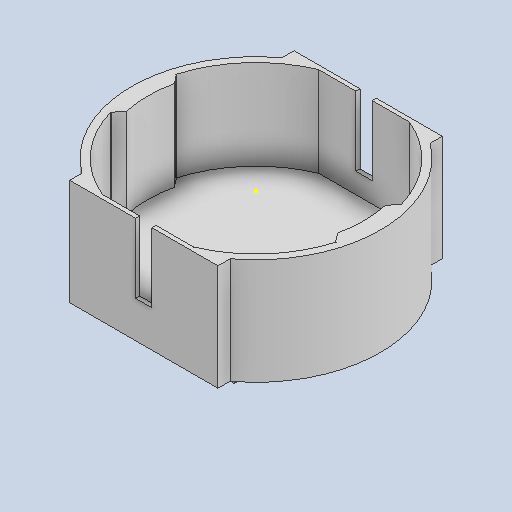
# Autodesk Inventor part: BigLif2
Saved by Autodesk Inventor 2025 (Build 290162000, 162)
## iProperties
Created: 2025-08-07
Part Number: BigLif2
Material: Generic
Document SubType Name: Modeling
Designer: Pravoslav
Density: 1 g/cm^3
Appearance: Default
Author: Pravoslav
Autodesk Inventor part; units mm, degrees
sketch "Sketch1" plane through (0, 0, 0) normal (0, 1, 0) x (-1, 0, 0)
  circle A0 centre (0, 0) radius 26.5
  circle A1 centre (0, 0) radius 30.5
  dimension "d0" = 53
  dimension "d1" = 4
  constraints: 2 centre point, 2 coincident
  measures "d0" diameter of A0
  measures "d1" radial gap between concentric circles of A0 A1
extrude "Extrusion1" add sketch "Sketch1" along normal blind 22
extrude "Extrusion2" add sketch "Sketch1" against normal blind 4 contours A0 | A1
ref_plane "Work Plane1" through (0, 15, 0) normal (0, 1, 0) x (1, 0, 0)
ref_plane "Work Plane2" through (30.5, 0, 0) normal (1, 0, 0) x (0, 1, 0)
sketch "Sketch3" plane through (30.5, 0, 0) normal (1, 0, 0) x (0, 1, 0)
  line L0 (14, -18.4883) -> (14, 18.4883) projected
  line L1 (16, 18.4883) -> (16, -18.4883) projected
  line L2 (16, 21.067) -> (16, 18.4883) projected
  line L3 (14, 18.4883) -> (14, 21.067) projected
  line L4 (16, 21.067) -> (16, -21.067) projected
  line L5 (16, 21.067) -> (16, 18.4883) projected
  line L6 (16, 18.4883) -> (16, -18.4883) projected
  line L7 (16, -18.4883) -> (16, -21.067) projected
  line L8 (14, -21.067) -> (14, -18.4883) projected
  line L9 (23, 32.2933) -> (-6, 32.2933)
  line L10 (-6, 32.2933) -> (-6, -38.454)
  line L11 (-6, -38.454) -> (23, -38.454)
  line L12 (23, -38.454) -> (23, 32.2933)
  line L13 (23, 24.5) -> (-6, 24.5)
  line L14 (23, -24.5) -> (-6.5731, -24.5)
  line L15 (-4, 30.5) -> (22, 30.5) projected
  line L16 (-4, -30.5) -> (22, -30.5) projected
  point P0 (0, 0)
  point P1 (-6, -24.5)
  dimension "d11" = 7
  dimension "d12" = 20
  dimension "d31" = 6
  dimension "d32" = 6
  constraints: 12 end point, 3 perpendicular, 3 point on line, 2 parallel, 1 horizontal
  measures "d11" distance between parallel lines of L1 L12
  measures "d12" distance between parallel lines of L3 L10
  measures "d31" distance between parallel lines of L15 L13
  measures "d32" distance between parallel lines of L14 L16
extrude "Extrusion4" cut sketch "Sketch3" against normal through all contours L12 L13 L10 L9 | L12 L11 L10 L14
sketch "Sketch4" plane through (0, 15, 0) normal (0, 1, 0) x (1, 0, 0)
  point P0 (0, 0)
ref_plane "Work Plane6" through (0, 0, 2) normal (0, 0, 1) x (1, 0, 0)
ref_plane "Work Plane5" through (0, 0, 30.5) normal (0, 0, 1) x (1, 0, 0)
sketch "Sketch6" plane through (0, 0, 2) normal (0, 0, 1) x (1, 0, 0)
  point P0 (0, 0)
sketch "Sketch7" plane through (0, 0, 2) normal (0, 0, 1) x (1, 0, 0)
  line L0 (-30.5, -4) -> (30.5, -4) projected
  line L1 (0, -4) -> (0, -71)
  circle A0 centre (0, -71) radius 57
  circle A1 centre (0, -71) radius 59.5
  circle A2 centre (0, -12.7932) radius 2.25
  circle A3 centre (-12.0008, -14) radius 2.25
  line L2 (4.6794, -4) -> (4.6794, -18.4597)
  line L3 (4.6794, -18.4597) -> (-15.0336, -19.4972)
  line L4 (-15.0336, -19.4972) -> (-17.1884, -4)
  point P0 (0, 0)
  dimension "d24" = 67
  dimension "d25" = 114
  dimension "d26" = 119
  dimension "d27" = 4.5
  dimension "d28" = 4.5
  constraints: 8 end point, 4 centre point, 3 point on line, 2 coincident, 2 vertical, 1 midpoint
  measures "d24" distance of L1.start L1.end
  measures "d25" diameter of A0
  measures "d26" diameter of A1
  measures "d27" diameter of A2
  measures "d28" diameter of A3
extrude "Extrusion6" add sketch "Sketch7" along normal mid plane 16 contours L0 L1 A2 A1 A3 L4 | L0 L2 A1 A2 L1 | A1 A3 A0 L4 | A0 A3 A2 L1 L3 L4 | L2 A0 A2 A1 | A2 A0 A3 A1 | L2 L3 L1 A2 A0
sketch "Sketch8" plane through (-18.1659, -4, 24.5) normal (0, 0, 1) x (1, 0, 0)
  line L0 (28.2654, 26) -> (36.3318, 26) projected
  line L1 (36.3318, 0) -> (0, 0) projected
  line L2 (36.3318, 26) -> (28.2654, 26)
  line L3 (28.2654, 26) -> (28.2654, 0)
  line L4 (28.2654, 0) -> (36.3318, 0)
  line L5 (36.3318, 0) -> (36.3318, 26)
  line L6 (28.2654, 4) -> (28.2654, 26) projected
  line L7 (0, 0) -> (0, 26) projected
  line L8 (36.3318, 0) -> (0, 0)
  line L9 (0, 0) -> (0, 4)
  line L10 (0, 4) -> (36.3318, 4)
  line L11 (36.3318, 4) -> (36.3318, 0)
  line L12 (8.0664, 26) -> (8.0664, 4) projected
  line L13 (0, 0) -> (8.0664, 0)
  line L14 (8.0664, 0) -> (8.0664, 26)
  line L15 (8.0664, 26) -> (0, 26)
  line L16 (0, 26) -> (0, 0)
  point P0 (18.1659, 4)
  dimension "d33" = 0
  constraints: 24 end point, 6 parallel, 3 horizontal, 3 perpendicular, 2 point on line
  measures "d33" distance between parallel lines of L3 L6
extrude "Extrusion7" add sketch "Sketch8" along normal blind 2
sketch "Sketch9" plane through (-18.1659, -4, 26.5) normal (0, 0, 1) x (1, 0, 0)
  line L0 (0, 0) -> (36.3318, 0) projected
  line L1 (8.0664, 26) -> (0, 26) projected
  line L2 (36.3318, 0) -> (0, 0)
  line L3 (0, 0) -> (0, 26)
  line L4 (0, 26) -> (36.3318, 26)
  line L5 (36.3318, 26) -> (36.3318, 0)
  line L6 (20.1659, 9) -> (16.1659, 9)
  line L7 (16.1659, 9) -> (16.1659, 26)
  line L8 (16.1659, 26) -> (20.1659, 26)
  line L9 (20.1659, 26) -> (20.1659, 9)
  line L10 (28.2654, 4) -> (8.0664, 4) projected
  point P0 (18.1659, 4)
  point P1 (18.1659, 4)
  point P2 (18.1659, 9)
  point P3 (18.1659, 4)
  dimension "d36" = 4
  dimension "d37" = 0
  dimension "d38" = 5
  dimension "d39" = 0
  constraints: 16 end point, 4 parallel, 3 midpoint, 2 horizontal, 2 perpendicular
  measures "d36" distance of L7.end L8.end
  measures "d37" horizontal distance of point (18.166, 4) point (18.166, 9)
  measures "d38" distance from line of point (18.166, 4) L6
  measures "d39" distance between parallel lines of L4 L8
extrude "Extrusion8" add sketch "Sketch9" along normal blind 1 contours L3 L1 L4 L7 L6 L9 L5 L0
mirror "Mirror1" about plane through (0, 0, 0) normal (0, 0, 1) of "Extrusion8", "Extrusion7"
sketch "Sketch10" plane through (0, 22, 0) normal (0, 1, 0) x (1, 0, 0)
  circle A0 centre (0, 0) radius 28.75
  line L0 (10.0995, -24.5) -> (10.0995, -26.5) projected
  line L1 (10.0995, -26.5) -> (11.74, -26.5)
  line L2 (10.0995, -26.5) -> (11.74, -26.5) construction
  line L3 (11.74, -26.5) -> (-11.1496, -26.5)
  line L4 (27.6145, -8) -> (-27.6145, -8)
  point P0 (0, -8)
  point P1 (11.1496, -26.5)
  dimension "d42" = 57.5
  dimension "d43" = 0
  dimension "d44" = 8
  constraints: 8 end point, 3 point on circle, 2 horizontal, 1 centre point, 1 coincident, 1 collinear, 1 midpoint, 1 point on line
  measures "d42" diameter of A0
  measures "d43" distance between parallel lines of L1 L2
  measures "d44" distance of point (0, 0) point (0, -8)
extrude "Extrusion9" cut sketch "Sketch10" against normal up to surface (22 mm away) contours L4 A0 L1 L3
chamfer "Chamfer1" distance 2.25 angle 45 2 edges at (-25.2636, 11, 8) (25.2636, 11, 8)
mirror "Mirror2" about plane through (0, 0, 0) normal (0, 0, 1) of "Extrusion9"
chamfer "Chamfer2" distance 2.25 angle 45 2 edges at (-25.2636, 11, -8) (25.2636, 11, -8)
ref_plane "Work Plane7" through (4.6794, -4, 1) normal (0.1736, -0.9848, 0) x (0, 0, -1)
sketch "Sketch11" plane through (4.6794, -4, 1) normal (0.1736, -0.9848, 0) x (0, 0, -1)
  line L0 (-26.5, -22.4982) -> (-26.5, 13.2817) projected
  line L1 (28.5, -22.4982) -> (28.5, 13.2817) projected
  line L2 (7, -2.5109) -> (-9, -2.5109) projected
  line L3 (-9, 0) -> (7, 0) projected
  circle A0 centre (1, 0) radius 2.15
  point P0 (1, -3.9137)
  dimension "d54" = 4.3
  dimension "d55" = 27.5
  constraints: 1 centre point, 1 point on line
  measures "d54" diameter of A0
  measures "d55" distance from line of L0 A0.centre
extrude "Extrusion10" cut sketch "Sketch11" along normal through all both and the other way through all
ref_plane "Work Plane3" through (30.5, 0, 0) normal (1, 0, 0) x (0, 1, 0)
sketch "Sketch5" plane through (2, 0, 0) normal (1, 0, 0) x (0, 1, 0)
  line L0 (-4, 30.5) -> (-4, -30.5) projected
  line L1 (-4, 0) -> (-71, 0)
  circle A0 centre (-71, 0) radius 57
  circle A1 centre (-71, 0) radius 59.5
  circle A2 centre (-12.675, 0) radius 1.5
  circle A3 centre (-14.6323, 14.7617) radius 1.5
  line L2 (-4, -4.4838) -> (-16.1323, -4.4838)
  line L3 (-16.1323, -4.4838) -> (-19.3598, 18.592)
  line L4 (-19.3598, 18.592) -> (-4, 18.9349)
  point P0 (0, 0)
  dimension "d16" = 67
  dimension "d17" = 114
  dimension "d18" = 119
  dimension "d19" = 3
  dimension "d20" = 3
  constraints: 8 end point, 4 centre point, 3 point on line, 2 coincident, 2 horizontal, 1 midpoint
  measures "d16" distance of L1.start L1.end
  measures "d17" diameter of A0
  measures "d18" diameter of A1
  measures "d19" diameter of A2
  measures "d20" diameter of A3
body "Solid1"
